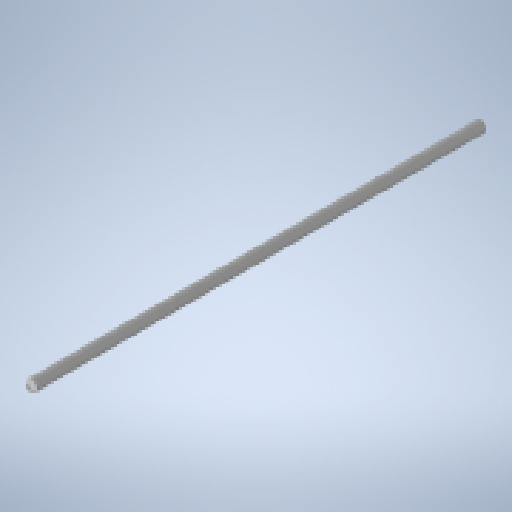
# Autodesk Inventor part: eixo_trapesoidal_001
Saved by Autodesk Inventor 2026 (Build 300175000, 175)
## iProperties
Created: 2025-04-10
Part Number: eixo_trapesoidal_001
Material: Generic
Document SubType Name: Modeling
Designer: Tony Dias
Density: 1 g/cm^3
Appearance: Default
Author: Tony Dias
Autodesk Inventor part; units mm, degrees
ref_plane "YZ Plane" through (0, 0, 0) normal (1, 0, 0) x (0, 1, 0)
ref_plane "XZ Plane" through (0, 0, 0) normal (0, 1, 0) x (-1, 0, 0)
ref_plane "XY Plane" through (0, 0, 0) normal (0, 0, 1) x (1, 0, 0)
sketch "Sketch1" plane through (0, 0, 0) normal (0, 0, 1) x (1, 0, 0)
  circle A0 centre (0, 0) radius 4
  dimension "d0" = 8
  constraints: 1 centre point, 1 coincident
  measures "d0" diameter of A0
extrude "Extrusion1" add sketch "Sketch1" along normal mid plane 320
thread "Thread1" size "M6x1" class "6g" standard "ANSI Metric M Profile" full length
chamfer "Chamfer1" distance 2 angle 45 2 edges at (-4, 0, 160) (-4, 0, -160)
body "Solid1"
